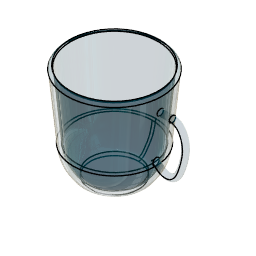
fabacademy cup (Autodesk Fusion 360 design; units mm, degrees)
Autodesk Fusion 360 part; units mm, degrees
sketch "Sketch1" plane through (0, 0, 0) normal (1, 0, 0) x (0, 1, 0)
  line L0 (0, 0) -> (76.165, 0)
  spline S0 degree 5 poles (76.165, 0) (77.7019, 0) (80.6604, 0.2185) (84.7519, 1.2015) (89.5486, 3.7231) (94.6399, 8.34) (99.0678, 13.7616) (103.0704, 19.3902) (106.8218, 24.9064) (110.4063, 30.3373) (113.847, 35.8937) (117.1208, 41.8633) (120.1769, 48.4942) (122.9554, 55.8554) (125.3949, 63.8601) (127.4356, 72.3411) (128.7074, 79.3515) (129.4411, 84.6634) (129.8304, 88.2188) (130, 90) knots 0 0 0 0 0 0 0.066667 0.133333 0.2 0.266667 0.333333 0.4 0.466667 0.533333 0.6 0.666667 0.733333 0.8 0.866667 0.933333 1 1 1 1 1 1
  line L1 (130, 90) -> (150, 300)
  line L2 (0, 11.4345) -> (76.165, 11.4345)
  spline S1 degree 3 poles (76.165, 11.4345) (77.9771, 11.4345) (79.2341, 11.7115) (80.4627, 12.2063) (81.6605, 12.6886) (82.8717, 13.4305) (84.2175, 14.5654) (86.1969, 16.2348) (88.3876, 18.7696) (90.576, 21.6779) (92.7703, 24.5941) (94.9734, 27.8143) (97.0717, 30.9405) (99.3833, 34.3844) (101.5606, 37.726) (103.5559, 41.1205) (105.6458, 44.676) (107.5563, 48.351) (109.3352, 52.5555) (111.3686, 57.3616) (113.2211, 62.8673) (114.7486, 68.8248) (116.3427, 75.0419) (117.5696, 81.6809) (118.3304, 88.3459) (118.4344, 89.2574) (118.5299, 90.1701) (118.617, 91.0841) knots 0 0 0 0 0.081739 0.081739 0.081739 0.16142 0.16142 0.16142 0.278617 0.278617 0.278617 0.396128 0.396128 0.396128 0.525576 0.525576 0.525576 0.66116 0.66116 0.66116 0.816145 0.816145 0.816145 0.977882 0.977882 0.977882 1 1 1 1
  line L3 (118.617, 91.0841) -> (138.617, 301.0841)
  line L4 (0, 0) -> (0, 11.4345)
  line L5 (138.617, 301.0841) -> (150, 300)
  point P0 (101.4592, 17.1805)
  point P1 (117.8774, 43.6841)
  dimension "d1" = -11.4345
  constraint coincident L0.start L4.start
  constraint horizontal L0
  constraint coincident S0.end L1.start
  constraint perpendicular L2 L4
  constraint perpendicular L1 L5
revolve "Revolve1" add sketch "Sketch1" angle 360 about axis through (0, 0, 1.75) along (0, 0, 1)
fillet "Fillet1" radius 10 2 edges at (-139.8491, 54.2423, 300) (-129.2364, 50.126, 301.0841)
sketch "Sketch2" plane through (0, 0, 0) normal (0, 1, 0) x (1, 0, 0)
  line L0 (137.9738, -244.5567) -> (182.505, -244.5567)
  spline S0 degree 5 poles (182.505, -244.5567) (184.0804, -244.458) (187.1575, -244.1354) (191.552, -243.275) (196.9684, -241.3743) (202.997, -237.7529) (208.2788, -232.9284) (212.8082, -226.9928) (216.5805, -220.1076) (219.5923, -212.5211) (221.8456, -204.5216) (223.3521, -196.3945) (224.1371, -188.3757) (224.2428, -180.6121) (223.7351, -173.1043) (222.6994, -165.7076) (221.2221, -158.212) (219.3761, -150.4013) (217.2041, -142.123) (214.704, -133.3487) (211.8095, -124.2508) (208.4159, -115.1529) (204.4119, -106.4635) (199.709, -98.618) (194.2739, -92.0145) (188.1542, -86.9577) (181.5217, -83.5843) (174.6544, -81.8564) (167.8642, -81.6172) (161.4379, -82.6291) (155.5785, -84.6172) (150.3313, -87.3133) (145.6171, -90.4739) (141.2955, -93.8903) (137.2136, -97.3999) (133.2701, -100.9018) (130.1875, -103.6579) (127.9083, -105.6919) (126.4035, -107.0332) (125.6548, -107.7002) knots 0 0 0 0 0 0 0.028571 0.057143 0.085714 0.114286 0.142857 0.171429 0.2 0.228571 0.257143 0.285714 0.314286 0.342857 0.371429 0.4 0.428571 0.457143 0.485714 0.514286 0.542857 0.571429 0.6 0.628571 0.657143 0.685714 0.714286 0.742857 0.771429 0.8 0.828571 0.857143 0.885714 0.914286 0.942857 0.971429 1 1 1 1 1 1
  point P0 (212.4358, -227.0362)
  point P1 (224.1161, -183.965)
  point P2 (216.8159, -140.8938)
  point P3 (191.2652, -89.7924)
  point P4 (160.2394, -83.2223)
  point P5 (140.1638, -94.9026)
  constraint horizontal L0
pipe "Pipe1" add diameter 20 path "Sketch2" along L0 S0
